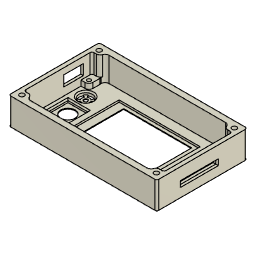
Display Mount - BTT TFT24 (Autodesk Fusion 360 design; units mm, degrees)
Autodesk Fusion 360 part; units mm, degrees
note: some values were not read from the file. Set by a fixed rule: which face or edge a step refers to.
sketch "Faceplate" plane through (0, 0, 0) normal (0, 1, 0) x (1, 0, 0)
  line L0 (52.5, 23) -> (-52.5, 23)
  line L1 (-52.5, 23) -> (-52.5, -23)
  line L2 (-52.5, -23) -> (52.5, -23)
  line L3 (52.5, -23) -> (52.5, 23)
  line L4 (52.5, 23) -> (-52.5, -23) construction
  line L5 (-52.5, 23) -> (52.5, -23) construction
  line L6 (50.4, 20.575) -> (-50.4, -20.575) construction
  line L7 (-50.4, 20.575) -> (50.4, -20.575) construction
  circle A0 centre (50.4, -20.575) radius 1.4
  circle A1 centre (-50.4, -20.575) radius 1.4
  circle A2 centre (50.4, 20.575) radius 1.4
  line L8 (53.5, 24) -> (-53.5, 24)
  line L9 (-53.5, 24) -> (-53.5, -24)
  line L10 (-53.5, -24) -> (53.5, -24)
  line L11 (53.5, -24) -> (53.5, 24)
  line L12 (-52.5, 23) -> (32.1, 23)
  line L13 (-52.5, 23) -> (-30.12, 23)
  line L14 (31.4, 21) -> (-29.82, 21)
  line L15 (-29.82, 21) -> (32.1, 21)
  line L16 (32.1, 21) -> (32.1, -21)
  line L17 (32.1, -21) -> (-29.82, -21)
  line L18 (-29.82, -21) -> (-29.82, 21)
  line L19 (32.1, 23) -> (32.1, 21)
  line L20 (56.5, 27) -> (-56.5, 27)
  line L21 (-56.5, 27) -> (-56.5, -27)
  line L22 (-56.5, -27) -> (56.5, -27)
  line L23 (56.5, -27) -> (56.5, 27)
  line L24 (-47.4, -20.575) -> (-47.4, -24)
  line L25 (-50.4, -17.575) -> (-53.5, -17.575)
  arc A3 (-47.4, -20.575) -> (-50.4, -17.575) centre (-50.4, -20.575) ccw
  line L26 (0, 23) -> (0, -23)
  line L27 (52.5, 0) -> (-52.5, 0)
  line L28 (-50.4, 17.575) -> (-53.5, 17.575)
  arc A4 (-50.4, 17.575) -> (-47.4, 20.575) centre (-50.4, 20.575) ccw
  line L29 (-47.4, 20.575) -> (-47.4, 24)
  circle A5 centre (-50.4, 20.575) radius 1.4
  line L30 (50.4, -17.575) -> (53.5, -17.575)
  arc A6 (50.4, -17.575) -> (47.4, -20.575) centre (50.4, -20.575) ccw
  line L31 (47.4, -20.575) -> (47.4, -24)
  circle A7 centre (50.4, -20.575) radius 1.4
  line L32 (47.4, 20.575) -> (47.4, 24)
  arc A8 (47.4, 20.575) -> (50.4, 17.575) centre (50.4, 20.575) ccw
  line L33 (50.4, 17.575) -> (53.5, 17.575)
  line L34 (28.1, 21) -> (28.1, -21)
  line L35 (-23.82, -21) -> (-23.82, 21)
  line L36 (-56.5, -27) -> (-56.5, -25)
  line L37 (-56.5, -27) -> (-54.5, -27)
  line L38 (-54.5, -27) -> (-56.5, -25)
  line L39 (56.5, -27) -> (56.5, -25)
  line L40 (56.5, -25) -> (54.5, -27)
  line L41 (56.5, 27) -> (56.5, 25)
  line L42 (56.5, 27) -> (54.5, 27)
  line L43 (54.5, 27) -> (56.5, 25)
  line L44 (-56.5, 27) -> (-54.5, 27)
  line L45 (-56.5, 27) -> (-56.5, 26.6653)
  line L46 (-56.5, 27) -> (-56.5, 25)
  line L47 (-56.5, 25) -> (-54.5, 27)
  line L48 (-29.82, -21) -> (32.1, -21)
  line L49 (32.1, -21) -> (32.1, -23)
  line L50 (32.1, -23) -> (-29.82, -23)
  line L51 (-29.82, -23) -> (-29.82, -21)
  line L52 (-29.82, 21) -> (32.1, 21)
  line L53 (32.1, 21) -> (32.1, 23)
  line L54 (32.1, 23) -> (-29.82, 23)
  line L55 (-29.82, 23) -> (-29.82, 21)
  dimension "d1" = 105
  dimension "d2" = 46
  dimension "d3" = 100.8
  dimension "d4" = 41.15
  dimension "d5" = 2.8
  dimension "d6" = 2.8
  dimension "d8" = 2.8
  dimension "d9" = 1
  dimension "d10" = 84.6
  dimension "d11" = 22.38
  dimension "d18" = 4
  dimension "d30" = 3
  dimension "d31" = 3
  dimension "d37" = 4
  dimension "d38" = 6
  dimension "d55" = 2
  dimension "d56" = 2
  dimension "d57" = 2
  dimension "d99" = 2
  constraint horizontal L0
  constraint perpendicular L0 L1
  constraint parallel L0 L2
  constraint parallel L1 L3
  constraint coincident L4 origin
  constraint coincident L5 origin
  constraint coincident L6 origin
  constraint coincident L7 origin
  constraint coincident L7.end A0.centre
  constraint coincident L6.end A1.centre
  constraint coincident L6.start A2.centre
  constraint perpendicular L1 L12
  constraint perpendicular L1 L13
  constraint horizontal L15
  constraint vertical L16
  constraint horizontal L17
  constraint vertical L18
  constraint perpendicular L15 L19
  constraint perpendicular L2 L24
  constraint perpendicular L1 L25
  constraint tangent L25 A3
  constraint midpoint L0 L26.start
  constraint midpoint L2 L26.end
  constraint midpoint L3 L27.start
  constraint midpoint L1 L27.end
  constraint symmetric A1 L27 A5
  constraint symmetric L25.start L27 L28.start
  constraint symmetric L24.start L27 A4.end
  constraint symmetric L24.end L27 L29.end
  constraint symmetric L25.end L27 L28.end
  constraint symmetric A3 L27 A4
  constraint symmetric A1 L26 A7
  constraint symmetric L25.start L26 L30.start
  constraint symmetric L24.start L26 A6.end
  constraint symmetric L24.end L26 L31.end
  constraint symmetric L25.end L26 L30.end
  constraint symmetric A3 L26 A6
  constraint symmetric L26 L28.start A8.end
  constraint symmetric L26 L28.end L33.end
  constraint symmetric L26 A4.end L32.start
  constraint symmetric L26 A4 A8
  constraint symmetric L26 L29.end L32.end
  constraint coincident L21 L36.end
  constraint perpendicular L22 L36
  constraint perpendicular L21 L37
  constraint coincident L23 L39.end
  constraint perpendicular L22 L39
  constraint coincident L22 L40.end
  constraint coincident L23 L41.end
  constraint perpendicular L20 L41
  constraint perpendicular L41 L42
  constraint perpendicular L21 L44
  constraint coincident L21 L45.end
  constraint coincident L21 L46.end
  constraint horizontal L48
  constraint vertical L49
  constraint horizontal L50
  constraint vertical L51
  constraint horizontal L52
  constraint vertical L53
  constraint horizontal L54
  constraint vertical L55
  measures "d1" distance of L1.end L2.end
  measures "d2" distance of L0.end L1.end
  measures "d3" distance of L6.end L7.end
  measures "d4" distance of L7.start L6.end
  measures "d5" diameter of A0
  measures "d6" diameter of A1
  measures "d8" diameter of A2
  measures "d10" distance of L0.end L12.end
  measures "d11" distance of L0.end L13.end
  measures "d30" distance of L6.end L25.start
  measures "d31" distance of L6.end L24.start
  measures "d55" distance of L21.end L37.end
  measures "d56" distance of L20.start L42.end
  measures "d57" distance of L20.end L44.end
  measures "d99" distance of L17.end L50.end
sketch "Buzzer" plane through (0, 0, 0) normal (0, 1, 0) x (-1, 0, 0)
  line L0 (52.5, 23) -> (-52.5, 23)
  line L1 (-52.5, 23) -> (-52.5, -23)
  line L2 (-52.5, -23) -> (52.5, -23)
  line L3 (52.5, -23) -> (52.5, 23)
  line L4 (52.5, 23) -> (-52.5, -23) construction
  line L5 (-52.5, 23) -> (52.5, -23) construction
  line L6 (52.5, 23) -> (44.69, 23)
  line L7 (44.69, 23) -> (44.69, 12.41)
  circle A0 centre (44.69, 12.41) radius 5.15
  dimension "d12" = 7.81
  dimension "d13" = 10.59
  dimension "d14" = 10.3
  constraint horizontal L0
  constraint perpendicular L0 L1
  constraint parallel L0 L2
  constraint parallel L1 L3
  constraint coincident L4 origin
  constraint coincident L5 origin
  constraint perpendicular L3 L6
  constraint perpendicular L0 L7
  constraint coincident L7.end A0.centre
  measures "d12" distance of L0.start L6.end
  measures "d13" distance of L6.end L7.end
  measures "d14" diameter of A0
sketch "Encoder" plane through (0, 0, 0) normal (0, 1, 0) x (1, 0, 0)
  line L0 (-52.5, -23) -> (-36.78, -23)
  line L1 (-36.78, -23) -> (-36.78, 9.08)
  line L2 (-36.78, -23) -> (-36.78, -2.09)
  line L3 (-36.78, 9.08) -> (-47.95, 9.08)
  line L4 (-36.78, -2.09) -> (-47.95, -2.09)
  line L5 (-47.95, 9.08) -> (-47.95, -2.09)
  line L6 (-36.78, -2.09) -> (-36.78, 9.08)
  line L7 (-34.78, -4.09) -> (-49.95, -4.09)
  line L8 (-49.95, 11.08) -> (-49.95, -4.09)
  line L9 (-34.78, 11.08) -> (-49.95, 11.08)
  line L10 (-34.78, -4.09) -> (-34.78, 11.08)
  circle A0 centre (-42.365, 3.495) radius 5
  dimension "d15" = 15.72
  dimension "d16" = 32.08
  dimension "d17" = 20.91
  dimension "d36" = 11.17
  dimension "d73" = 2
  dimension "d83" = 10
  constraint horizontal L0
  constraint perpendicular L0 L1
  constraint perpendicular L0 L2
  constraint perpendicular L1 L3
  constraint perpendicular L2 L4
  constraint perpendicular L4 L5
  measures "d15" distance of L0.start L0.end
  measures "d16" distance of L0.end L1.end
  measures "d17" distance of L0.end L2.end
  measures "d36" distance of L1.end L3.end
  measures "d83" diameter of A0
extrude "Extrude1" add sketch "Buzzer" sketch "Encoder" sketch "Faceplate" along normal blind 3 of sketch 2 contours L1 L3 L4 L5 L6 | A0 of sketch 3 contours L0 L8 L12 L13 L29 L32 L54 | L0 L3 L8 L11 L32 L33 | L14 L15 L16 L27 L34 L52 | L14 L15 L26 L27 L35 L52 | L14 L15 L26 L27 L34 L52 | L16 L17 L27 L34 L48 | L14 L15 L18 L27 L35 L52 | L17 L26 L27 L34 L48 | L17 L26 L27 L35 L48 | L3 L11 L30 L33 | L0 L1 L8 L9 L12 L13 L28 L29 | L17 L18 L27 L35 L48 | L2 L10 L24 L31 L50 | L2 L3 L10 L11 L30 L31 | L1 L9 L25 L28 | L1 L2 L9 L10 L24 L25 | A0 A7 | A1 | A2 | L20 L23 L41 L42 L43 | L20 L21 L22 L23 L38 L40 L43 L47 | L20 L21 L44 L45 L46 L47 | L22 L23 L39 L40 | L21 L22 L36 L37 L38 makes body 1
extrude "Extrude2" cut sketch "Encoder" along normal blind 3 contours A0 bodies 1
extrude "Extrude3" cut sketch "Faceplate" along normal blind 3 contours L14 L15 L16 L27 L34 L52 | L14 L15 L26 L27 L35 L52 | L14 L15 L26 L27 L34 L52 | L16 L17 L27 L34 L48 | L14 L15 L18 L27 L35 L52 | L17 L26 L27 L34 L48 | L17 L26 L27 L35 L48 | L17 L18 L27 L35 L48 bodies 1
sketch "Reset Button" plane through (0, 0, 0) normal (0, 1, 0) x (-1, 0, 0)
  line L0 (52.5, 23) -> (-52.5, 23)
  line L1 (-52.5, 23) -> (-52.5, -23)
  line L2 (-52.5, -23) -> (52.5, -23)
  line L3 (52.5, -23) -> (52.5, 23)
  line L4 (52.5, 23) -> (-52.5, -23) construction
  line L5 (-52.5, 23) -> (52.5, -23) construction
  line L6 (52.5, -23) -> (52.5, -19.31)
  line L7 (52.5, -19.31) -> (39.04, -19.31)
  circle A0 centre (39.04, -19.31) radius 2.25
  dimension "d25" = 3.69
  dimension "d26" = 13.46
  dimension "d27" = 4.5
  constraint horizontal L0
  constraint perpendicular L0 L1
  constraint parallel L0 L2
  constraint parallel L1 L3
  constraint coincident L4 origin
  constraint coincident L5 origin
  constraint perpendicular L2 L6
  constraint perpendicular L6 L7
  constraint coincident L7.end A0.centre
  measures "d25" distance of L2.end L6.end
  measures "d26" distance of L6.end L7.end
  measures "d27" diameter of A0
extrude "Extrude4" cut sketch "Reset Button" along normal blind 3 contours A0 bodies 1
extrude "Extrude5" add sketch "Faceplate" against normal blind 4 contours L0 L3 L8 L11 L32 L33 | L0 L3 L32 A8 L33 | L0 L1 L8 L9 L12 L13 L28 L29 | L0 L1 L12 L13 L28 A4 L29 | L2 L3 L10 L11 L30 L31 | L2 L3 L30 A6 L31 | L1 L2 L24 L25 A3 | L1 L2 L9 L10 L24 L25 bodies 1
extrude "Extrude6" add sketch "Faceplate" against normal blind 6 contours L20 L23 L41 L42 L43 | L20 L21 L22 L23 L38 L40 L43 L47 | L20 L21 L44 L45 L46 L47 | L22 L23 L39 L40 | L21 L22 L36 L37 L38 bodies 1
extrude "Extrude7" add sketch "Faceplate" along normal blind 3 contours L14 L15 L16 L27 L34 L52 | L16 L17 L27 L34 L48 | L14 L15 L18 L27 L35 L52 | L17 L18 L27 L35 L48 bodies 1
ref_plane "WorkPlane1" through (0, -6, 0) normal (0, -1, 0) x (0, 0, -1)
extrude "Extrude8" add 1 faces at (-17.8333, -6, -26) along direction (0, -1, 0) blind 12.7 separate body on bodies 1 makes body 2
sketch "USB Port" plane through (-53.5, 0, 0) normal (1, 0, 0) x (0, 1, 0)
  line L0 (-6, -24) -> (-6, 24)
  line L1 (-6, 24) -> (-18.7, 24)
  line L2 (-18.7, 24) -> (-18.7, -24)
  line L3 (-18.7, -24) -> (-6, -24)
  line L4 (-6, 24) -> (-6, 19.4)
  line L5 (-6, 19.4) -> (-14, 19.4)
  line L6 (-14, 19.4) -> (-14, 4.4)
  line L7 (-14, 4.4) -> (-6, 4.4)
  line L8 (-6, 4.4) -> (-6, 19.4)
  dimension "d44" = 4.6
  dimension "d45" = 15
  constraint coincident L0.end L1.start
  constraint perpendicular L1 L4
  constraint perpendicular L0 L5
  constraint perpendicular L5 L6
  constraint coincident L0 L7.end
  constraint perpendicular L0 L7
  measures "d44" distance of L0.end L4.end
  measures "d45" distance of L5.end L6.end
sketch "SD Card" plane through (53.5, 0, 0) normal (-1, 0, 0) x (0, -1, 0)
  line L0 (6, 24) -> (6, -24)
  line L1 (6, -24) -> (18.7, -24)
  line L2 (18.7, -24) -> (18.7, 24)
  line L3 (18.7, 24) -> (6, 24)
  line L4 (6, -24) -> (6, -15.5)
  line L5 (6, -15.5) -> (8.5, -15.5)
  line L6 (8.5, -15.5) -> (6, -15.5)
  line L7 (6, -15.5) -> (6, 11.5)
  line L8 (6, 11.5) -> (8.5, 11.5)
  line L9 (8.5, 11.5) -> (8.5, -15.5)
  dimension "d48" = 8.5
  dimension "d49" = 2.5
  dimension "d50" = 27
  constraint coincident L0.end L1.start
  constraint perpendicular L1 L4
  constraint perpendicular L4 L5
  constraint horizontal L6
  constraint vertical L7
  constraint horizontal L8
  constraint vertical L9
  measures "d48" distance of L0.end L4.end
  measures "d49" distance of L4.end L5.end
  measures "d50" distance of L5.end L8.end
combine "Combine1" operation add target body 1 tool bodies 2
fillet "Fillet2" radius 1.5 4 edges at (53.5, -11.35, 24) (-53.5, -11.35, 24) (-53.5, -11.35, -24) (53.5, -11.35, -24) on bodies 1
move_face "OffsetFaces1" offset -2 1 faces at (15.8, -13.8, 24) on bodies 1
move_face "OffsetFaces2" offset -2 1 faces at (-15.8, -13.8, -24) on bodies 1
sketch "Buzzer Cover" plane through (-44.69, 3, 12.41) normal (0, 1, 0) x (-1, 0, 0)
  circle A0 centre (0, 0) radius 1.5
  circle A1 centre (0, 0) radius 3
  line L0 (0, 0) -> (0, 3)
  line L1 (0, 0) -> (3, 0) construction
  circle A2 centre (0, 0) radius 5.25
  circle A3 centre (0, 0) radius 5.15
  line L2 (-20.87, -33.41) -> (-72.79, -33.41)
  line L3 (-72.79, -33.41) -> (-72.79, 8.59)
  line L4 (-72.79, 8.59) -> (-20.87, 8.59)
  line L5 (-20.87, 8.59) -> (-20.87, -33.41)
  circle A4 centre (-5.65, -31.72) radius 2.25
  line L6 (0, 0) -> (3, 0) construction
  line L7 (-1.5, 2.5981) -> (-2.5756, 4.4611)
  line L8 (-1.5, 2.5981) -> (0.6512, 2.5981) construction
  line L9 (1.5, 2.5981) -> (2.575, 4.46)
  line L10 (1.5, 2.5981) -> (3.65, 2.5981) construction
  line L11 (-2.5981, 1.5) -> (-4.46, 2.575)
  line L12 (-2.5981, -1.5) -> (-4.4611, -2.5756)
  line L13 (-1.5, -2.5981) -> (-2.575, -4.46)
  line L14 (1.5, -2.5981) -> (2.5756, -4.4611)
  line L15 (2.5981, -1.5) -> (4.46, -2.575)
  line L16 (2.5981, 1.5) -> (4.4611, 2.5756)
  circle A5 centre (-2.325, -15.905) radius 5
  line L17 (-101.19, 14.59) -> (-101.19, -39.41)
  line L18 (-101.19, -39.41) -> (11.81, -39.41)
  line L19 (11.81, -39.41) -> (11.81, 14.59)
  line L20 (11.81, 14.59) -> (-101.19, 14.59)
  dimension "d63" = 3
  dimension "d64" = 6
  dimension "d67" = 10.5
  dimension "d77" = 120
  dimension "d78" = 60
  dimension "d80" = 360
  constraint coincident A0.centre A1.centre
  constraint coincident A1 L0.end
  constraint vertical L0
  constraint horizontal L1
  constraint concentric A1 A2
  constraint horizontal L6
  constraint horizontal L8
  constraint horizontal L10
  constraint coincident A3 L9.end
  measures "d63" diameter of A0
  measures "d64" diameter of A1
  measures "d67" diameter of A2
  measures "d77" angle of L7 L8
  measures "d78" angle of L9 L10
sketch "Panel" plane through (0, -18.7, 0) normal (0, -1, 0) x (1, 0, 0)
  line L0 (-53.5, -23) -> (-53.5, 23)
  arc A0 (-52, 24.5) -> (-53.5, 23) centre (-52, 23) ccw
  line L1 (-52, 24.5) -> (52, 24.5)
  arc A1 (53.5, 23) -> (52, 24.5) centre (52, 23) ccw
  line L2 (53.5, 23) -> (53.5, -23)
  arc A2 (52, -24.5) -> (53.5, -23) centre (52, -23) ccw
  line L3 (52, -24.5) -> (-52, -24.5)
  arc A3 (-53.5, -23) -> (-52, -24.5) centre (-52, -23) ccw
  arc A4 (55, -27) -> (56.5, -25.5) centre (55, -25.5) ccw
  line L4 (56.5, -25.5) -> (56.5, 25.5)
  arc A5 (56.5, 25.5) -> (55, 27) centre (55, 25.5) ccw
  line L5 (55, 27) -> (-55, 27)
  arc A6 (-55, 27) -> (-56.5, 25.5) centre (-55, 25.5) ccw
  line L6 (-56.5, 25.5) -> (-56.5, -25.5)
  arc A7 (-56.5, -25.5) -> (-55, -27) centre (-55, -25.5) ccw
  line L7 (-55, -27) -> (55, -27)
  line L8 (56.5, -27) -> (-56.5, 27) construction
  line L9 (-56.5, -27) -> (56.5, 27) construction
  line L10 (-55, 34.5) -> (55, 34.5)
  arc A8 (-55, 34.5) -> (-56.5, 33) centre (-55, 33) ccw
  arc A9 (56.5, 33) -> (55, 34.5) centre (55, 33) ccw
  circle A10 centre (-51.5, 29.5) radius 1.8
  circle A11 centre (51.5, 29.75) radius 1.8
  line L11 (56.5, 0) -> (-56.5, 0)
  line L12 (-56.5, 33) -> (-56.5, 25.5)
  line L13 (56.5, 33) -> (56.5, 25.5)
  line L14 (-56.5, -33) -> (-56.5, -25.5)
  line L15 (-55, -34.5) -> (55, -34.5)
  arc A12 (-56.5, -33) -> (-55, -34.5) centre (-55, -33) ccw
  circle A13 centre (-51.5, -29.5) radius 1.8
  circle A14 centre (51.5, -29.75) radius 1.8
  arc A15 (55, -34.5) -> (56.5, -33) centre (55, -33) ccw
  line L16 (56.5, -33) -> (56.5, -25.5)
  line L17 (-53.5, -23) -> (-53.5, 23)
  arc A16 (-52, 24.5) -> (-53.5, 23) centre (-52, 23) ccw
  line L18 (-52, 24.5) -> (52, 24.5)
  arc A17 (53.5, 23) -> (52, 24.5) centre (52, 23) ccw
  line L19 (53.5, 23) -> (53.5, -23)
  arc A18 (52, -24.5) -> (53.5, -23) centre (52, -23) ccw
  line L20 (52, -24.5) -> (-52, -24.5)
  arc A19 (-53.5, -23) -> (-52, -24.5) centre (-52, -23) ccw
  arc A20 (55, -27) -> (56.5, -25.5) centre (55, -25.5) ccw
  line L21 (56.5, -25.5) -> (56.5, 25.5)
  arc A21 (56.5, 25.5) -> (55, 27) centre (55, 25.5) ccw
  line L22 (55, 27) -> (-55, 27)
  arc A22 (-55, 27) -> (-56.5, 25.5) centre (-55, 25.5) ccw
  line L23 (-56.5, 25.5) -> (-56.5, -25.5)
  arc A23 (-56.5, -25.5) -> (-55, -27) centre (-55, -25.5) ccw
  line L24 (-55, -27) -> (55, -27)
  line L25 (-53.5, -23) -> (-53.5, 23)
  arc A24 (-52, 24.5) -> (-53.5, 23) centre (-52, 23) ccw
  line L26 (-52, 24.5) -> (52, 24.5)
  arc A25 (53.5, 23) -> (52, 24.5) centre (52, 23) ccw
  line L27 (53.5, 23) -> (53.5, -23)
  arc A26 (52, -24.5) -> (53.5, -23) centre (52, -23) ccw
  line L28 (52, -24.5) -> (-52, -24.5)
  arc A27 (-53.5, -23) -> (-52, -24.5) centre (-52, -23) ccw
  arc A28 (55, -27) -> (56.5, -25.5) centre (55, -25.5) ccw
  line L29 (56.5, -25.5) -> (56.5, 25.5)
  arc A29 (56.5, 25.5) -> (55, 27) centre (55, 25.5) ccw
  line L30 (55, 27) -> (-55, 27)
  arc A30 (-55, 27) -> (-56.5, 25.5) centre (-55, 25.5) ccw
  line L31 (-56.5, 25.5) -> (-56.5, -25.5)
  arc A31 (-56.5, -25.5) -> (-55, -27) centre (-55, -25.5) ccw
  line L32 (-55, -27) -> (55, -27)
  line L33 (-53.5, -23) -> (-53.5, 23)
  arc A32 (-52, 24.5) -> (-53.5, 23) centre (-52, 23) ccw
  line L34 (-52, 24.5) -> (52, 24.5)
  arc A33 (53.5, 23) -> (52, 24.5) centre (52, 23) ccw
  line L35 (53.5, 23) -> (53.5, -23)
  arc A34 (52, -24.5) -> (53.5, -23) centre (52, -23) ccw
  line L36 (52, -24.5) -> (-52, -24.5)
  arc A35 (-53.5, -23) -> (-52, -24.5) centre (-52, -23) ccw
  arc A36 (55, -27) -> (56.5, -25.5) centre (55, -25.5) ccw
  line L37 (56.5, -25.5) -> (56.5, 25.5)
  arc A37 (56.5, 25.5) -> (55, 27) centre (55, 25.5) ccw
  line L38 (55, 27) -> (-55, 27)
  arc A38 (-55, 27) -> (-56.5, 25.5) centre (-55, 25.5) ccw
  line L39 (-56.5, 25.5) -> (-56.5, -25.5)
  arc A39 (-56.5, -25.5) -> (-55, -27) centre (-55, -25.5) ccw
  line L40 (-55, -27) -> (55, -27)
  line L41 (-53.5, -24.5) -> (-53.5, 23)
  arc A40 (-52, 24.5) -> (-53.5, 23) centre (-52, 23) ccw
  line L42 (-52, 24.5) -> (52, 24.5)
  arc A41 (53.5, 23) -> (52, 24.5) centre (52, 23) ccw
  line L43 (53.5, 23) -> (53.5, -24.5)
  arc A42 (52, -26) -> (53.5, -24.5) centre (52, -24.5) ccw
  line L44 (52, -26) -> (-52, -26)
  arc A43 (-53.5, -24.5) -> (-52, -26) centre (-52, -24.5) ccw
  line L45 (56.5, -27) -> (56.5, 27)
  line L46 (56.5, 27) -> (-56.5, 27)
  line L47 (-56.5, 27) -> (-56.5, -27)
  line L48 (-56.5, -27) -> (56.5, -27)
  line L49 (-53.5, -24.5) -> (-53.5, 24.5)
  arc A44 (-52, 26) -> (-53.5, 24.5) centre (-52, 24.5) ccw
  line L50 (-52, 26) -> (52, 26)
  arc A45 (53.5, 24.5) -> (52, 26) centre (52, 24.5) ccw
  line L51 (53.5, 24.5) -> (53.5, -24.5)
  arc A46 (52, -26) -> (53.5, -24.5) centre (52, -24.5) ccw
  line L52 (52, -26) -> (-52, -26)
  arc A47 (-53.5, -24.5) -> (-52, -26) centre (-52, -24.5) ccw
  line L53 (56.5, -27) -> (56.5, 27)
  line L54 (56.5, 27) -> (-56.5, 27)
  line L55 (-56.5, 27) -> (-56.5, -27)
  line L56 (-56.5, -27) -> (56.5, -27)
  line L57 (-56.5, -27) -> (-47.5, -27)
  line L58 (-47.5, -27) -> (-47.5, -30)
  line L59 (56.5, -27) -> (47.5, -27)
  line L60 (47.5, -27) -> (47.5, -30)
  line L61 (47.5, -30) -> (-47.5, -30)
  line L62 (-47.5, 27) -> (-47.5, 30)
  line L63 (47.5, 30) -> (-47.5, 30)
  line L64 (47.5, 27) -> (47.5, 30)
  line L65 (-47.5, -27) -> (-47.5, -26)
  line L66 (47.5, -27) -> (47.5, -26)
  line L67 (47.5, 27) -> (47.5, 26)
  line L68 (-47.5, 27) -> (-47.5, 26)
  dimension "d84" = 113
  dimension "d85" = 54
  dimension "d88" = 3.6
  dimension "d92" = 3.6
  dimension "d110" = 9
  dimension "d111" = 9
  constraint coincident L8 origin
  constraint coincident L9 origin
  constraint tangent L10 A8
  constraint midpoint L4 L11.start
  constraint coincident A6.end L6.start
  constraint tangent A6 L12
  constraint coincident L4.end A5.start
  constraint tangent A5 L13
  constraint symmetric A8.end L11 L14.start
  constraint symmetric A9.start L11 A15.end
  constraint symmetric L10.end L11 L15.end
  constraint symmetric L10.start L11 L15.start
  constraint symmetric A8 L11 A12
  constraint symmetric A9 L11 A15
  constraint symmetric A10 L11 A13
  constraint symmetric A11 L11 A14
  constraint symmetric L11 A6.end L6.end
  constraint symmetric L11 L4.end A4.end
  constraint parallel L56 L57
  constraint perpendicular L57 L58
  constraint perpendicular L45 L59
  constraint perpendicular L59 L60
  constraint perpendicular L58 L61
  constraint symmetric L11 L57.end L62.start
  constraint symmetric L11 L58.end L62.end
  constraint symmetric L11 L59.end L64.start
  constraint symmetric L11 L60.end L63.start
  constraint coincident L44 L65.end
  constraint perpendicular L44 L65
  constraint coincident L44 L66.end
  constraint perpendicular L44 L66
  constraint coincident L50 L67.end
  constraint perpendicular L50 L67
  constraint coincident L50 L68.end
  constraint perpendicular L50 L68
  measures "d84" distance of L8.end L9.end
  measures "d85" distance of L9.start L8.end
  measures "d88" diameter of A10
  measures "d92" diameter of A11
  measures "d110" distance of L9.start L57.end
  measures "d111" distance of L8.start L59.end
extrude "Extrude14" add sketch "Panel" against normal blind 21.7 separate body contours L0 L6 A7 L7 L11 L17 L23 A23 L24 L25 L31 A31 L32 L33 L39 A39 L40 L41 L44 A43 L47 L48 L49 L52 A47 L55 L56 L57 L65 | L0 L5 A6 L6 L11 L17 L22 A22 L23 L25 L30 A30 L31 L33 L38 A38 L39 L41 L46 L47 L49 A44 L50 L54 L55 L68 | L2 A4 L4 L7 L11 L19 A20 L21 L24 L27 A28 L29 L32 L35 A36 L37 L40 L43 A42 L44 L45 L48 L51 A46 L52 L53 L56 L59 L66 | L2 L4 A5 L5 L11 L19 L21 A21 L22 L27 L29 A29 L30 L35 L37 A37 L38 L43 L45 L46 L50 A45 L51 L53 L54 L67 | A6 L12 A22 A30 A38 L46 L47 L54 L55 | A7 L14 A23 A31 A39 L47 L48 L55 L56 L57 | L7 L24 L32 L40 L44 L48 L52 L56 L65 L66 | A4 L16 A20 A28 A36 L45 L48 L53 L56 L59 | A5 L13 A21 A29 A37 L45 L46 L53 L54 | L5 L10 A8 A9 L12 L13 L22 L30 L38 L46 L54 L62 L63 L64 | L7 L14 L15 A12 A15 L16 L24 L32 L40 L48 L56 L57 L58 L59 L60 L61 | L7 L24 L32 L40 L48 L56 L58 L60 L61 | L5 L22 L30 L38 L46 L50 L54 L67 L68 | L5 L22 L30 L38 L46 L54 L62 L63 L64 | A10 | A11 | A13 | A14 makes body 3
combine "Combine2" operation add target body 1 tool bodies 3
extrude "Extrude12" add sketch "Buzzer Cover" against normal blind 0.6 contours A1 | A1 A3 L9 L16 | A1 A3 L14 L15 | A1 A3 L12 L13 | A1 A3 L7 L11 bodies 1
extrude "Extrude9" cut sketch "USB Port" against normal blind 3 contours L0 L5 L6 L7 L8 bodies 1
extrude "Extrude10" cut sketch "SD Card" against normal blind 3 contours L0 L5 L6 L7 L8 L9 bodies 1
extrude "Extrude11" cut sketch "Faceplate" along normal blind 1.5 contours L0 L12 L14 L15 L19 L26 L52 L53 L54 | L0 L12 L14 L15 L26 L52 L54 L55 | L14 L15 L16 L27 L34 L52 | L16 L17 L27 L34 L48 | L14 L15 L18 L27 L35 L52 | L2 L17 L26 L48 L49 L50 | L17 L18 L27 L35 L48 | L2 L17 L26 L48 L50 L51 bodies 1
extrude "Extrude13" cut sketch "Encoder" along normal blind 3 contours L1 L3 L4 L5 L6 | L7 L8 L9 L10 bodies 1
chamfer "Chamfer1" distance 1 angle 45 4 edges at (-56.5, -10, 19.4) (-56.5, -6, 11.9) (-56.5, -10, 4.4) (-56.5, -14, 11.9) on bodies 1
chamfer "Chamfer2" distance 1 angle 45 4 edges at (56.5, -8.5, -2) (56.5, -7.25, 11.5) (56.5, -6, -2) (56.5, -7.25, -15.5) on bodies 1
chamfer "Chamfer3" distance 1 angle 45 4 edges at (2.14, 3, 21) (-23.82, 3, 0) (2.14, 3, -21) (28.1, 3, 0) on bodies 1
chamfer "Chamfer4" distance 1 angle 45 6 edges at (-39.8885, 0, 14.2723) (-36.9423, 0, -20.1236) (-34.78, 0, -3.495) (-42.365, 0, 4.09) (-49.95, 0, -3.495) (-42.365, 0, -11.08) on bodies 1
move_face "OffsetFaces4" offset 1.5 1 faces at (-6.5133, 1.6667, -21) on bodies 1
move_face "OffsetFaces5" offset 0.5 1 faces at (10.7933, 1.6667, 21) on bodies 1
sketch "Encoder Cover" plane through (0, 3, 0) normal (0, 1, 0) x (-1, 0, 0)
  circle A0 centre (39.04, -19.31) radius 2.25
  line L0 (42.115, 7.95) -> (43.19, 9.8119)
  arc A1 (43.19, 9.8119) -> (46.19, 9.8119) centre (44.69, 12.41) ccw
  line L1 (46.19, 9.8119) -> (47.265, 7.95)
  arc A2 (42.115, 7.95) -> (47.265, 7.95) centre (44.69, 12.41) ccw
  circle A3 centre (44.69, 12.41) radius 1.5
  line L2 (40.23, 14.985) -> (42.0919, 13.91)
  arc A4 (42.0919, 13.91) -> (42.0919, 10.91) centre (44.69, 12.41) ccw
  line L3 (42.0919, 10.91) -> (40.23, 9.835)
  arc A5 (40.23, 14.985) -> (40.23, 9.835) centre (44.69, 12.41) ccw
  line L4 (47.265, 16.87) -> (46.19, 15.0081)
  arc A6 (46.19, 15.0081) -> (43.19, 15.0081) centre (44.69, 12.41) ccw
  line L5 (43.19, 15.0081) -> (42.115, 16.87)
  arc A7 (47.265, 16.87) -> (42.115, 16.87) centre (44.69, 12.41) ccw
  arc A8 (49.15, 9.835) -> (49.15, 14.985) centre (44.69, 12.41) ccw
  line L6 (49.15, 9.835) -> (47.2881, 10.91)
  arc A9 (47.2881, 10.91) -> (47.2881, 13.91) centre (44.69, 12.41) ccw
  line L7 (47.2881, 13.91) -> (49.15, 14.985)
  line L8 (34.78, 4.09) -> (49.95, 4.09)
  line L9 (49.95, 4.09) -> (49.95, -11.08)
  line L10 (49.95, -11.08) -> (34.78, -11.08)
  line L11 (34.78, -11.08) -> (34.78, 4.09)
  circle A10 centre (42.365, -3.495) radius 5.5
  line L12 (-56.5, 33) -> (-56.5, -33)
  arc A11 (-56.5, -33) -> (-55, -34.5) centre (-55, -33) ccw
  line L13 (-55, -34.5) -> (55, -34.5)
  arc A12 (55, -34.5) -> (56.5, -33) centre (55, -33) ccw
  line L14 (56.5, -33) -> (56.5, 33)
  arc A13 (56.5, 33) -> (55, 34.5) centre (55, 33) ccw
  line L15 (55, 34.5) -> (-55, 34.5)
  arc A14 (-55, 34.5) -> (-56.5, 33) centre (-55, 33) ccw
  line L16 (24.82, 21.5) -> (24.82, -20.5)
  line L17 (24.82, -20.5) -> (-29.1, -20.5)
  line L18 (-29.1, -20.5) -> (-29.1, 21.5)
  line L19 (-29.1, 21.5) -> (24.82, 21.5)
  line L20 (34.78, 4.09) -> (49.95, 4.09)
  line L21 (49.95, 4.09) -> (49.95, -11.08)
  line L22 (49.95, -11.08) -> (34.78, -11.08)
  line L23 (34.78, -11.08) -> (34.78, 4.09)
  dimension "d103" = 11
  constraint horizontal L8
  constraint vertical L9
  constraint horizontal L10
  constraint vertical L11
  measures "d103" diameter of A10
extrude "Extrude16" add sketch "Encoder Cover" against normal blind 0.6 contours L8 L9 L10 L11 L20 L21 L22 L23 bodies 1
extrude "Extrude17" cut sketch "Panel" against normal blind 6 contours A10 | A11 | A13 | A14 bodies 1
extrude "Extrude18" cut sketch "Panel" against normal up to surface (18.7 mm away) contours L7 L24 L32 L40 L44 L48 L52 L56 L65 L66 | L7 L24 L32 L40 L48 L56 L58 L60 L61 | L5 L22 L30 L38 L46 L50 L54 L67 L68 | L5 L22 L30 L38 L46 L54 L62 L63 L64 bodies 1
fillet "Fillet4" radius 3 8 edges at (-47.5, -9.35, -30) (-47.5, -11.35, -26) (-47.5, -9.35, 30) (-47.5, -11.35, 26) (47.5, -11.35, 26) (47.5, -9.35, 30) (47.5, -11.35, -26) (47.5, -9.35, -30) on bodies 1
move_body "Move1" bodies 1 to x (1, 0, 0) y (0, 0, -1) z (0, 1, 0) at (0, 15.8, -53.2)
chamfer "Chamfer5" distance 1.2 angle 45 8 edges at (0, -18.7, -56.2) (-56.0607, -18.2607, -56.2) (-56.5, 15.8, -56.2) (-56.0607, 49.8607, -56.2) (0, 50.3, -56.2) (56.0607, 49.8607, -56.2) (56.5, 15.8, -56.2) (56.0607, -18.2607, -56.2) on bodies 1
equation "d13 = 6.09 mm + 4.5 mm"
named bodies: "TFT24 Case"
